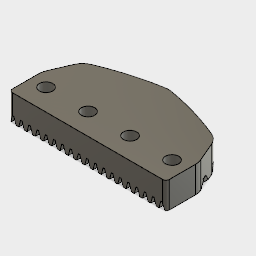
Gear Rack v3 (Autodesk Fusion 360 design; units mm, degrees)
Autodesk Fusion 360 part; units mm, degrees
sketch "Sketch1" plane through (0, 0, 0) normal (0, 1, 0) x (1, 0, 0)
  line L0 (-31.6667, 0) -> (31.6667, 0)
  line L1 (-31.6667, 0) -> (-31.6667, -38)
  line L2 (-31.6667, -38) -> (31.6667, -38)
  line L3 (31.6667, -38) -> (31.6667, 0)
  line L4 (-31.6667, -6.5) -> (31.6667, -6.5)
  arc A0 (31.6667, -6.5) -> (31.6667, 6.5) centre (31.6667, 0) ccw
  line L5 (31.6667, 6.5) -> (-31.6667, 6.5)
  arc A1 (-31.6667, 6.5) -> (-31.6667, -6.5) centre (-31.6667, 0) ccw
  line L6 (-31.6667, 0) -> (31.6667, 0) construction
  line L7 (31.6667, -31.5) -> (-31.6667, -31.5)
  arc A2 (-31.6667, -31.5) -> (-31.6667, -44.5) centre (-31.6667, -38) ccw
  line L8 (-31.6667, -44.5) -> (31.6667, -44.5)
  arc A3 (31.6667, -44.5) -> (31.6667, -31.5) centre (31.6667, -38) ccw
  line L9 (31.6667, -38) -> (-31.6667, -38) construction
  line L10 (-38.1667, 0) -> (-38.1667, -38)
  arc A4 (-38.1667, -38) -> (-25.1667, -38) centre (-31.6667, -38) ccw
  line L11 (-25.1667, -38) -> (-25.1667, 0)
  arc A5 (-25.1667, 0) -> (-38.1667, 0) centre (-31.6667, 0) ccw
  line L12 (-31.6667, 0) -> (-31.6667, -38) construction
  line L13 (25.1667, -38) -> (25.1667, 0)
  arc A6 (25.1667, 0) -> (38.1667, 0) centre (31.6667, 0) ccw
  line L14 (38.1667, 0) -> (38.1667, -38)
  arc A7 (38.1667, -38) -> (25.1667, -38) centre (31.6667, -38) ccw
  line L15 (31.6667, -38) -> (31.6667, 0) construction
  line L16 (10.5, -16.5) -> (-10.5, -16.5)
  line L17 (-10.5, -16.5) -> (-10.5, 16.5)
  line L18 (-10.5, 16.5) -> (10.5, 16.5)
  line L19 (10.5, 16.5) -> (10.5, -16.5)
  line L20 (10.5, -16.5) -> (-10.5, 16.5) construction
  line L21 (-10.5, -16.5) -> (10.5, 16.5) construction
  line L22 (7, -24.5) -> (-7, -24.5)
  line L23 (-7, -24.5) -> (-7, -8.5)
  line L24 (-7, -8.5) -> (7, -8.5)
  line L25 (7, -8.5) -> (7, -24.5)
  line L26 (7, -24.5) -> (-7, -8.5) construction
  line L27 (-7, -24.5) -> (7, -8.5) construction
  line L28 (0, -38) -> (0, -20)
  line L29 (8, -38) -> (8, -22.5)
  line L30 (4, -38) -> (4, -21)
  line L31 (12, -38) -> (12, -22.5)
  line L32 (16, -38) -> (16, -24)
  line L33 (20, -38) -> (20, -26)
  line L34 (23, -38) -> (23, -33)
  arc A8 (20, -26) -> (0, -20) centre (-12.7912, -98.9708) ccw
  line L35 (20, -26) -> (25.1429, -38)
  point P0 (0, -16.5)
  dimension "d1" = 63.3333
  dimension "d2" = 38
  dimension "d3" = 13
  dimension "d4" = 10
  dimension "d5" = 21
  dimension "d6" = 14
  dimension "d7" = 8
  dimension "d10" = 4
  dimension "d11" = 4
  dimension "d12" = 4
  dimension "d13" = 4
  dimension "d14" = 4
  dimension "d15" = 18
  dimension "d16" = 15.5
  dimension "d17" = 17
  dimension "d18" = 15.5
  dimension "d19" = 14
  dimension "d20" = 12
  dimension "d21" = 5
  dimension "d22" = 3
  dimension "d23" = 80
  measures "d1" distance of L0.start L0.end
  measures "d2" distance of L0.start L1.end
  measures "d3" distance of L7 L8
  measures "d4" distance of L4 L16
  measures "d5" distance of L17 L19
  measures "d6" distance of L22.start L22.end
  measures "d7" distance of L16 L22
  measures "d10" distance of L28 L30
  measures "d11" distance of L29 L30
  measures "d12" distance of L29 L31
  measures "d13" distance of L31 L32
  measures "d14" distance of L32 L33
  measures "d15" distance of L28.start L28.end
  measures "d16" distance of L31.start L31.end
  measures "d17" distance of L30.start L30.end
  measures "d18" distance of L29.start L29.end
  measures "d19" distance of L32.start L32.end
  measures "d20" distance of L33.start L33.end
  measures "d21" distance of L34.start L34.end
  measures "d22" distance of L33 L34
  measures "d23" radius of A8
sketch "Sketch2" plane through (0, 0, 0) normal (0, 1, 0) x (1, 0, 0)
  arc A0 (20, -26) -> (0, -20) centre (-12.7912, -98.9708) ccw
  line L0 (20, -26) -> (25.1429, -38)
  arc A1 (0, -20) -> (-20, -26) centre (12.7912, -98.9708) ccw
  line L1 (-20, -26) -> (-25.1429, -38)
  line L2 (23.6667, -34.5556) -> (23.6667, -44.5)
  line L3 (23.6667, -44.5) -> (-23.6667, -44.5)
  line L4 (-23.6667, -44.5) -> (-23.6667, -34.5556)
  line L5 (0, 0) -> (0, -20) construction
  line L6 (-31.6667, -44.5) -> (31.6667, -44.5)
  arc A2 (-38.1667, -38) -> (-25.1667, -38) centre (-31.6667, -38) ccw
  line L7 (-31.6667, -38) -> (23.6667, -38) construction
  circle A3 centre (-19, -38) radius 2
  circle A4 centre (19, -38) radius 2
  circle A5 centre (-6.3333, -38) radius 2
  circle A6 centre (6.3333, -38) radius 2
  line L8 (-6.3333, -38) -> (-19, -38)
  line L9 (-19, -38) -> (-6.3333, -38)
  line L10 (-6.3333, -38) -> (6.3333, -38)
  line L11 (6.3333, -38) -> (19, -38)
  dimension "d24" = 8
  dimension "d25" = 38
  dimension "d26" = 4
  measures "d24" distance of L4 A2.centre
  measures "d25" distance of A3.centre A4.centre
  measures "d26" diameter of A3
extrude "Extrude1" add sketch "Sketch2" along normal blind 12
sketch "Sketch3" plane through (0, 12, 0) normal (0, 1, 0) x (-1, 0, 0)
  circle A0 centre (6.3333, 38) radius 2
  circle A1 centre (19, 38) radius 2
  circle A2 centre (-19, 38) radius 2
  circle A3 centre (-6.3333, 38) radius 2
  arc A4 (-20, 26) -> (0, 20) centre (12.7912, 98.9708) ccw
  arc A5 (0, 20) -> (20, 26) centre (-12.7912, 98.9708) ccw
  line L0 (20, 26) -> (23.6667, 34.5556)
  line L1 (23.6667, 34.5556) -> (23.6667, 44.5)
  line L2 (23.6667, 44.5) -> (-23.6667, 44.5)
  line L3 (-23.6667, 44.5) -> (-23.6667, 34.5556)
  line L4 (-23.6667, 34.5556) -> (-20, 26)
  line L5 (23.6667, 44.5) -> (-23.6667, 44.5)
  line L6 (-23.6667, 44.5) -> (-23.6667, 31)
  line L7 (-23.6667, 31) -> (23.6667, 31)
  line L8 (23.6667, 31) -> (23.6667, 44.5)
  dimension "d29" = 13.5
  measures "d29" distance of L2.end L6.end
extrude "Extrude2" cut sketch "Sketch3" against normal blind 4 contours L0 L1 L2 L3 L4 L5 L6 L7 L8
sketch "Sketch4" plane through (0, 0, 44.5) normal (0, 0, 1) x (1, 0, 0)
  line L0 (23.6667, 8) -> (-23.6667, 8)
  line L1 (-23.6667, 8) -> (-23.6667, 0)
  line L2 (-23.6667, 0) -> (23.6667, 0)
  line L3 (23.6667, 0) -> (23.6667, 8)
  line L4 (-0.8127, 0) -> (-0.2863, 2)
  line L5 (-0.2863, 2) -> (0.1629, 2)
  line L6 (0.1629, 2) -> (0.8127, 0)
  line L7 (-0.8127, 0) -> (0.8127, 0)
  dimension "d32" = 0.4492
  dimension "d34" = 2
  dimension "d36" = 72
  measures "d32" distance of L4.end L5.end
  measures "d34" distance of L5 L7
  measures "d36" angle of L5 L6
extrude "Extrude3" cut sketch "Sketch4" against normal blind 38 contours L2 L4 L5 L6 L7
pattern_linear "R-Pattern1" count 20 spacing 2.487 along (-1, 0, 0) both ways of "Extrude3"
fillet "Fillet1" radius 5 5 edges at (0, 7, 20) (20, 7, 26) (-20, 7, 26) (-23.6667, 4, 34.5556) (23.6667, 4, 34.5556)
fillet "Fillet2" radius 0.5 1 edges at (0, 8, 31)
fillet "Fillet3" radius 2 1 edges at (0, 12, 31)
fillet "Fillet4" radius 2 1 edges at (0, 8, 44.5)
fillet "Fillet5" radius 1 23 edges at (-23.6667, 3, 44.5) (-23.6667, 7.4142, 43.9142) (-23.6667, 8, 39.0409) (-23.5646, 8, 34.5765) (-22.8098, 8, 32.5561) (-22.2056, 8.1464, 31.1464) (-22.1429, 9.25, 31) (-21.8918, 11.4142, 30.4142) (-21.034, 12, 28.4127) (-19.7076, 12, 26.245) (-9.6277, 12, 22.1763) (0, 12, 20.0696) (9.6277, 12, 22.1763) (19.7076, 12, 26.245) (21.034, 12, 28.4127) (21.8918, 11.4142, 30.4142) (22.1429, 9.25, 31) (22.2056, 8.1464, 31.1464) (22.8098, 8, 32.5561) (23.5646, 8, 34.5765) (23.6667, 8, 39.0409) (23.6667, 7.4142, 43.9142) (23.6667, 3, 44.5)
sketch "Sketch5" plane through (0, 8, 0) normal (0, 1, 0) x (-1, 0, 0)
  circle A0 centre (19, 38) radius 2
  circle A1 centre (-6.3333, 38) radius 2
  circle A2 centre (-19, 38) radius 2
  circle A3 centre (6.3333, 38) radius 2
  line L0 (-22.6667, 42.5) -> (-22.6667, 35.5818)
  arc A4 (-22.6667, 35.5818) -> (-22.3432, 34.0062) centre (-18.6667, 35.5818) ccw
  line L1 (-22.3432, 34.0062) -> (-21.2692, 31.5)
  line L2 (-21.2692, 31.5) -> (21.2692, 31.5)
  line L3 (21.2692, 31.5) -> (22.3432, 34.0062)
  arc A5 (22.3432, 34.0062) -> (22.6667, 35.5818) centre (18.6667, 35.5818) ccw
  line L4 (22.6667, 35.5818) -> (22.6667, 42.5)
  line L5 (22.6667, 42.5) -> (-22.6667, 42.5)
  line L6 (-21.8062, 32.7531) -> (21.8062, 32.7531)
  line L7 (21.8062, 32.7531) -> (21.8062, 20)
  line L8 (21.8062, 20) -> (-22, 20)
  line L9 (-22, 20) -> (-21.8062, 32.7531)
extrude "Extrude4" cut sketch "Sketch5" along normal through all contours L1 L2 L3 L7 L8 L9
delete_face "DeleteFace1" 13 faces at (-22.1157, 7.5599, 31.3718) (-22.6914, 7.7071, 33.0235) (-22.08, 7.2149, 30.9036) (-23.3294, 7.1893, 33.8273) (-22.7142, 7.9989, 37.8879) (-22.8559, 7.9618, 42.7821) (-7.5556, 7.9909, 42.6901) (21.6297, 7.9142, 30.9221) (21.8687, 7.8286, 31.4777) (22.6914, 7.7071, 33.0235) (23.5231, 7.1893, 34.4706) (23.1249, 7.8888, 40.1939) (22.9484, 7.9241, 42.8708)
